rod_label_collar (Autodesk Fusion 360 design; units mm, degrees)
part number: 2026-09-06-10-05-05-328
Autodesk Fusion 360 part; units mm, degrees
sketch "Lips" plane through (0, 0, 0) normal (0, 1, 0) x (1, 0, 0)
  circle A0 centre (0, 0) radius 17.05
  circle A1 centre (0, 0) radius 19.45
  dimension "d78" = 34.1
  dimension "d79" = 38.9
  constraint coincident A0.centre A1.centre
  constraint concentric A0 A1
  measures "d78" diameter of A0
  measures "d79" diameter of A1
extrude "Lips (1)" add sketch "Lips" along normal blind 11.8 and the other way blind 8.2
sketch "Band" plane through (0, 0, 0) normal (0, 1, 0) x (1, 0, 0)
  circle A0 centre (0, 0) radius 17.05
  circle A1 centre (0, 0) radius 22
  dimension "d84" = 34.1
  dimension "d85" = 44
  constraint coincident A0.centre A1.centre
  constraint concentric A0 A1
  measures "d84" diameter of A0
  measures "d85" diameter of A1
extrude "Band (1)" add sketch "Band" along normal blind 8.1941 and the other way blind 7.2
sketch "Outer cone profile" plane through (0, 0, 0) normal (0, 0, 1) x (1, 0, 0)
  line L0 (0, 1.75) -> (0, 22.5) construction
  line L1 (1.75, 0) -> (22.5, 0) construction
  line L2 (22, 5.6441) -> (22, 8.1941)
  line L3 (22, 8.1941) -> (19.45, 8.1941)
  line L4 (19.45, 8.1941) -> (22, 5.6441)
  dimension "d90" = 22
  dimension "d91" = 19.45
  dimension "d92" = 5.6441
  dimension "d93" = 8.1941
  constraint parallel L0 L2
  constraint parallel L1 L3
  measures "d90" distance of L0 L2.start
  measures "d91" distance of L0 L3.end
  measures "d92" distance of L1 L2.start
  measures "d93" distance of L1 L3.end
revolve "Outer cone" cut sketch "Outer cone profile" angle 360 about axis through (0, 1.75, 0) along (0, 1, 0)
sketch "Pocket profile" plane through (0, 0, 0) normal (0, 0, 1) x (1, 0, 0)
  line L0 (0, 1.75) -> (0, 22.5) construction
  line L1 (1.75, 0) -> (22.5, 0) construction
  line L2 (0, -7.2) -> (17.05, -7.2)
  line L3 (17.05, -7.2) -> (19.6, -4.65)
  line L4 (19.6, -4.65) -> (19.6, 4.65)
  line L5 (19.6, 4.65) -> (17.05, 7.2)
  line L6 (17.05, 7.2) -> (0, 7.2)
  line L7 (0, 7.2) -> (0, -7.2)
  dimension "d95" = 17.05
  dimension "d96" = 19.6
  dimension "d97" = 7.2
  dimension "d98" = 4.65
  constraint coincident L0 L2.start
  constraint parallel L1 L2
  constraint symmetric L1 L2.start L6.end
  constraint symmetric L1 L2.end L5.end
  constraint symmetric L1 L3.end L4.end
  measures "d95" distance of L0 L2.end
  measures "d96" distance of L0 L3.end
  measures "d97" distance of L1 L2.end
  measures "d98" distance of L1 L3.end
revolve "Pocket" cut sketch "Pocket profile" angle 360 about axis through (0, 1.75, 0) along (0, 1, 0)
sketch "Mouth" plane through (0, 0, 0) normal (0, 1, 0) x (1, 0, 0)
  line L0 (0, 0) -> (46.7654, -27)
  line L1 (46.7654, -27) -> (0, -54)
  line L2 (0, -54) -> (-46.7654, -27)
  line L3 (-46.7654, -27) -> (0, 0)
  line L4 (0, 0) -> (0, -54) construction
  dimension "d100" = 54
  dimension "d101" = 54
  dimension "d102" = 54
  dimension "d103" = 60
  dimension "d104" = 60
  constraint coincident L0.start L3.end
  constraint vertical L4
  constraint coincident L1.end L2.start
  measures "d100" distance of L0.start L0.end
  measures "d101" distance of L0.start L2.end
  measures "d102" distance of L0.start L1.end
  measures "d103" angle of L0 L4
  measures "d104" angle of L3 L4
extrude "Mouth (1)" cut sketch "Mouth" along normal mid plane 30
ref_plane "WorkPlane3" through (0, 12.125, 0) normal (-0.173648, 0, -0.984808) x (0, 1, 0)
sketch "Stem slot section" plane through (0, 0, 0) normal (-0.173648, 0, -0.984808) x (0, 1, 0)
  line L0 (1.75, 0) -> (22.5, 0) construction
  line L1 (-4.65, 1.5) -> (4.65, 1.5)
  line L2 (4.65, 1.5) -> (4.65, -1.5)
  line L3 (4.65, -1.5) -> (-4.65, -1.5)
  line L4 (-4.65, -1.5) -> (-4.65, 1.5)
  line L5 (0, 0) -> (0, 4.8) construction
  dimension "d109" = 4.8
  dimension "d110" = 3
  dimension "d111" = 9.3
  constraint parallel L0 L1
  constraint parallel L0 L3
  constraint perpendicular L0 L4
  constraint perpendicular L0 L2
  constraint symmetric L0 L1 L3
  constraint coincident L5.start origin
  constraint perpendicular L0 L5
  constraint symmetric L2 L4 L5
  measures "d109" distance of L5.start L5.end
  measures "d110" distance of L1 L3
  measures "d111" distance of L2 L4
extrude "Stem slot" cut sketch "Stem slot section" along normal blind 6.4 from surface at 18.6
equation "rodOuterDiameter = 33.4 mm" comment "rod the collar snaps onto"
equation "collarClearance = 0.7 mm" comment "diametral, so it slides"
equation "collarWall = 2.4 mm" comment "wall thickness everywhere"
equation "collarWidth = 20.0 mm" comment "total width along the rod"
equation "mouthHalfAngleDeg = 60.0 deg" comment "half the mouth opening"
equation "ringOuterDiameter = 38.9 mm" comment "clip ring OD retrofitted"
equation "ringWidth = 9.0 mm" comment "clip ring width retrofitted"
equation "stemThickness = 2.4 mm" comment "clip stem thickness"
equation "stemAngleDeg = 100.0 deg" comment "clip stem angle below horizontal"
equation "pocketClearance = 0.3 mm" comment "over the ring, dia and width"
equation "slotClearance = 0.6 mm" comment "total across the stem"
equation "pocketWidth = ringWidth + pocketClearance" comment "derived: pocket width"
equation "pocketChamfer = ( ringOuterDiameter + pocketClearance ) / 2 - ( rodOuterDiameter + collarClearance ) / 2" comment "derived: 45 deg ledge, pocket bore to rod bore"
equation "bandWidth = pocketWidth + 2 * pocketChamfer" comment "derived: band over the pocket and its chamfers"
equation "farLip = 1.0 mm" comment "bearing land beyond the far ledge"
equation "farExtent = bandWidth / 2 + farLip" comment "derived: far end of the collar from the ring centre"
equation "chamferShift = collarWall * ( sqrt(2) - 1 )" comment "derived: outer cone offset that keeps the wall full thickness"
equation "d78 = rodOuterDiameter + collarClearance"
equation "d79 = rodOuterDiameter + collarClearance + 2 * collarWall"
equation "d80 = collarWidth - farExtent"
equation "d82 = farExtent"
equation "d84 = rodOuterDiameter + collarClearance"
equation "d85 = ringOuterDiameter + pocketClearance + 2 * collarWall"
equation "d86 = bandWidth / 2 + chamferShift"
equation "d88 = bandWidth / 2"
equation "d90 = ( ringOuterDiameter + pocketClearance + 2 * collarWall ) / 2"
equation "d91 = ( rodOuterDiameter + collarClearance + 2 * collarWall ) / 2"
equation "d92 = pocketWidth / 2 + chamferShift"
equation "d93 = bandWidth / 2 + chamferShift"
equation "d95 = ( rodOuterDiameter + collarClearance ) / 2"
equation "d96 = ( ringOuterDiameter + pocketClearance ) / 2"
equation "d97 = bandWidth / 2"
equation "d98 = pocketWidth / 2"
equation "d100 = ( ( ringOuterDiameter + pocketClearance + 2 * collarWall ) / 2 + 5 mm ) / cos(mouthHalfAngleDeg)"
equation "d101 = ( ( ringOuterDiameter + pocketClearance + 2 * collarWall ) / 2 + 5 mm ) / cos(mouthHalfAngleDeg)"
equation "d102 = ( ( ringOuterDiameter + pocketClearance + 2 * collarWall ) / 2 + 5 mm ) / cos(mouthHalfAngleDeg)"
equation "d103 = mouthHalfAngleDeg"
equation "d104 = mouthHalfAngleDeg"
equation "d105 = collarWidth + 10 mm"
equation "d107 = stemAngleDeg"
equation "d109 = stemThickness * 2"
equation "d110 = stemThickness + slotClearance"
equation "d111 = pocketWidth"
equation "d112 = ( ringOuterDiameter + pocketClearance ) / 2 - 1 mm"
equation "d113 = ( ringOuterDiameter + pocketClearance + 2 * collarWall ) / 2 - ( ringOuterDiameter + pocketClearance ) / 2 + 4 mm"
named bodies: "rod_label_collar"
